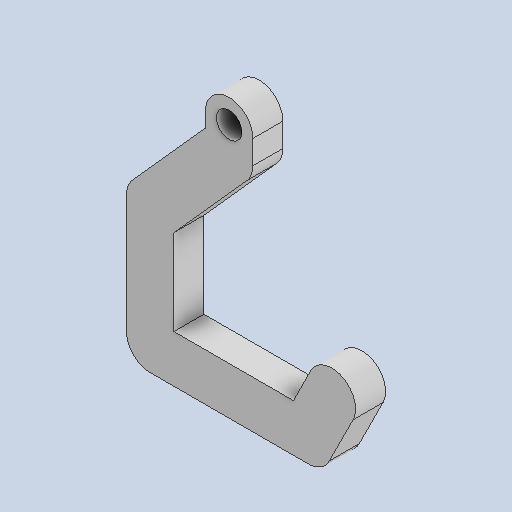
# Autodesk Inventor part: carlig 2
Saved by Autodesk Inventor 2025.2 (Build 292293000, 293)
## iProperties
Created: 2025-04-08
Part Number: carlig 2
Material: Generic
Document SubType Name: Modeling
Designer: mirewn
Density: 1 g/cm^3
Appearance: Default
Author: mirewn
Autodesk Inventor part; units mm, degrees
ref_plane "YZ Plane" through (0, 0, 0) normal (1, 0, 0) x (0, 1, 0)
ref_plane "XZ Plane" through (0, 0, 0) normal (0, 1, 0) x (-1, 0, 0)
ref_plane "XY Plane" through (0, 0, 0) normal (0, 0, 1) x (1, 0, 0)
sketch "Sketch1" plane through (0, 0, 0) normal (0, 0, 1) x (1, 0, 0)
  circle A0 centre (0, 0) radius 1.6
  arc A1 (3, 0) -> (-3, 0) centre (0, 0) ccw
  line L0 (-3, 0) -> (-3, -1.8541)
  line L1 (-3, -3) -> (3, -3) construction
  line L2 (3, -3) -> (3, 0)
  arc A2 (-2.2361, -1) -> (-3, -3) centre (0, -3) ccw construction
  arc A3 (-13, -29.1803) -> (-10, -32.1803) centre (-10, -29.1803) ccw
  arc A4 (7, -29.1803) -> (12.6833, -30.522) centre (10, -29.1803) ccw
  arc A5 (15.6833, -24.522) -> (10.3167, -21.8387) centre (13, -23.1803) ccw
  arc A6 (-12.2361, -12.1803) -> (-13, -14.1803) centre (-10, -14.1803) ccw
  line L3 (-10, -29.1803) -> (10, -29.1803) construction
  line L4 (-7.7639, -16.1803) -> (-7, -15.3262)
  line L5 (-12.2361, -12.1803) -> (-3, -1.8541)
  line L6 (-13, -14.1803) -> (-13, -29.1803)
  line L7 (-7, -14.1803) -> (-7, -15.3262)
  line L8 (-10, -26.1803) -> (-7, -26.1803)
  line L9 (-10, -32.1803) -> (10, -32.1803)
  line L10 (10.3167, -21.8387) -> (7.3167, -27.8387)
  line L11 (12.6833, -30.522) -> (15.6833, -24.522)
  line L12 (-3, -1.8541) -> (-2.2361, -1) construction
  arc A7 (3, -3) -> (-2.2361, -1) centre (0, -3) ccw
  arc A8 (-3, -3) -> (2.2361, -5) centre (0, -3) ccw construction
  line L13 (-3, -1.8541) -> (-3, -3) construction
  arc A9 (2.2361, -5) -> (3, -3) centre (0, -3) ccw
  line L14 (-7, -15.3262) -> (2.2361, -5)
  line L15 (-7, -15.3262) -> (-7, -26.1803)
  arc A10 (-13, -14.1803) -> (-7, -14.1803) centre (-10, -14.1803) ccw construction
  line L16 (-7, -26.1803) -> (10, -26.1803)
  line L17 (-7, -26.1803) -> (-7, -29.1803)
  arc A11 (-10, -26.1803) -> (-13, -29.1803) centre (-10, -29.1803) ccw construction
  arc A12 (-10, -32.1803) -> (-10, -26.1803) centre (-10, -29.1803) ccw construction
  arc A13 (7.3167, -27.8387) -> (7, -29.1803) centre (10, -29.1803) ccw construction
  arc A14 (10, -26.1803) -> (7.3167, -27.8387) centre (10, -29.1803) ccw construction
  arc A15 (12.6833, -30.522) -> (10, -26.1803) centre (10, -29.1803) ccw construction
  arc A16 (10.3167, -21.8387) -> (15.6833, -24.522) centre (13, -23.1803) ccw construction
  point P0 (0, -29.1803)
  point P1 (8.1459, -26.1803)
  dimension "d0" = 3.2
  dimension "d1" = 6
  dimension "d2" = 3
  dimension "d3" = 6
  dimension "d4" = 6
  dimension "d5" = 6
  dimension "d6" = 6
  dimension "d7" = 15
  dimension "d8" = 6
  dimension "d9" = 15
  dimension "d10" = 20
  dimension "d11" = 3
  dimension "d12" = 6
  constraints: 53 tangent, 39 point on circle, 36 end point, 17 centre point, 5 vertical, 3 vertical alignment, 2 coincident, 2 midpoint, 2 point on line, 1 horizontal alignment
  measures "d0" diameter of A0
  measures "d1" diameter of A1
  measures "d2" distance of L0.start L1.start
  measures "d3" diameter of A3
  measures "d4" diameter of A4
  measures "d5" diameter of A5
  measures "d6" diameter of A6
  measures "d7" distance of A6.centre A2.centre
  measures "d8" diameter of A2
  measures "d9" distance of L3.start A6.centre
  measures "d10" distance of L3.end L3.start
  measures "d11" horizontal distance of L3.end A5.centre
  measures "d12" vertical distance of L3.end A5.centre
extrude "Extrusion1" add sketch "Sketch1" along normal blind 3.8
body "Solid1"
